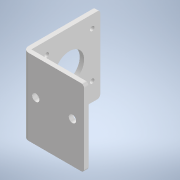
# Autodesk Inventor part: YAufnahmeMotor
Saved by Autodesk Inventor 2021 (Build 250183000, 183)
## iProperties
Created: 2020-01-07
Part Number: YAufnahmeMotor
Material: Generisch
Document SubType Name: Modeling
Designer: kaebi
Density: 1 g/cm^3
Appearance: Vorgabe
Description: Aufnahme x-Motor (Bestand)
Stock Number: -
Author: kaebi
Autodesk Inventor part; units mm, degrees
ref_plane "YZ Plane" through (0, 0, 0) normal (1, 0, 0) x (0, 1, 0)
ref_plane "XZ Plane" through (0, 0, 0) normal (0, 1, 0) x (-1, 0, 0)
ref_plane "XY Plane" through (0, 0, 0) normal (0, 0, 1) x (1, 0, 0)
sketch "Skizze1" plane through (0, 0, 0) normal (0, 1, 0) x (-1, 0, 0)
  line L0 (0, -50) -> (0, -4)
  line L1 (-4, 0) -> (-42, 0)
  line L2 (-42, 0) -> (-42, -3)
  line L3 (-42, -3) -> (-3, -3)
  line L4 (-3, -3) -> (-3, -50)
  line L5 (-3, -50) -> (0, -50)
  arc A0 (0, -4) -> (-4, 0) centre (-4, -4) ccw
  line L6 (0, -60.1657) -> (0, 10.9941) projected
  line L7 (9.3941, 0) -> (-50.5657, 0) projected
  point P0 (0, 0)
  point P1 (0, 0)
  dimension "d0" = 42
  dimension "d1" = 50
  dimension "d2" = 3
  dimension "d3" = 4
  constraints: 12 end point, 4 perpendicular, 2 collinear, 2 point on circle, 2 point on line, 2 tangent, 2 vertical, 1 centre point, 1 parallel
  measures "d0" distance of point (0, 0) L1.end
  measures "d1" distance of L0.start point (0, 0)
  measures "d2" distance of L1.end L2.end
  measures "d3" radius of A0
extrude "Extrusion1" add sketch "Skizze1" along normal mid plane 52 contours L5 L4 L3 L2 L1 A0 L0
fillet "Rundung1" radius 2 4 edges at (1.5, 26, -50) (1.5, -26, -50) (42, 26, -1.5) (42, -26, -1.5)
sketch "Skizze2" plane through (4, -26, 0) normal (0, 0, 1) x (1, 0, 0)
  circle A0 centre (5, 28) radius 2.5
  circle A1 centre (30, 28) radius 2.5
  line L0 (38, 2) -> (38, 50) projected
  line L1 (-166, 18) -> (204, 18) projected
  line L2 (-1, 0) -> (36, 0) projected
  line L3 (204, 18) -> (-166, 18) projected
  point P0 (-4, 26)
  point P1 (38, 26)
  dimension "d7" = 5
  dimension "d8" = 8
  dimension "d9" = 25
  dimension "d25" = 10
  dimension "d26" = 10
  constraints: 2 centre point, 1 equal radius, 1 midpoint
  measures "d7" diameter of A1
  measures "d8" distance from line of L0 A1.centre
  measures "d9" distance of A0.centre A1.centre
  measures "d25" distance from line of L3 A1.centre
  measures "d26" distance from line of L3 A0.centre
extrude "Extrusion2" cut sketch "Skizze2" against normal through all
sketch "Skizze3" plane through (0, -26, -4) normal (-1, 0, 0) x (0, 0, 1)
  circle A0 centre (-40.5, 43.5) radius 1.5
  circle A1 centre (-9.5, 43.5) radius 1.5
  circle A2 centre (-9.5, 12.5) radius 1.5
  circle A3 centre (-40.5, 12.5) radius 1.5
  circle A4 centre (-25, 28) radius 10
  line L0 (-46, 50) -> (-46, 2) projected
  line L1 (-25, 41.9808) -> (-25, 15.4808)
  circle A5 centre (-25, 28) radius 2.5 projected
  point P0 (4, 26)
  dimension "d12" = 31
  dimension "d13" = 31
  dimension "d14" = 3
  dimension "d16" = 20
  dimension "d21" = 15.5
  dimension "d22" = 31
  constraints: 5 centre point, 3 equal radius, 2 end point, 2 horizontal alignment, 1 concentric, 1 point on line, 1 vertical, 1 vertical alignment, 1 other
  measures "d12" distance of A1.centre A0.centre
  measures "d13" distance of A0.centre A3.centre
  measures "d14" diameter of A0
  measures "d16" diameter of A4
  measures "d21" horizontal distance of A0.centre A4.centre
  measures "d22" distance of A2.centre A3.centre
extrude "Extrusion3" cut sketch "Skizze3" against normal through all
